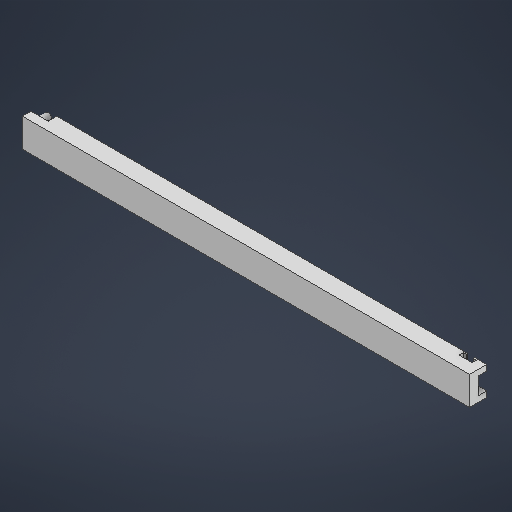
# Autodesk Inventor part: Wiper-supportipt
Saved by Autodesk Inventor 2026.2 (Build 302298010, 298A)
## iProperties
Created: 2026-06-02
Part Number: Wiper-supportipt
Material: Genérico
Document SubType Name: Modeling
Designer: pauli
Density: 1 g/cm^3
Appearance: Padrão
Author: pauli
Autodesk Inventor part; units mm, degrees
ref_plane "YZ Plane" through (0, 0, 0) normal (1, 0, 0) x (0, 1, 0)
ref_plane "XZ Plane" through (0, 0, 0) normal (0, 1, 0) x (-1, 0, 0)
ref_plane "XY Plane" through (0, 0, 0) normal (0, 0, 1) x (1, 0, 0)
sketch "Esboço1" plane through (0, 0, 0) normal (0, 0, 1) x (1, 0, 0)
  circle A0 centre (0, 0) radius 1.2
  line L0 (0, 0) -> (0, 4.75) construction
  circle A1 centre (0, 4.75) radius 1.2
  dimension "d0" = 2.4
  dimension "d1" = 4.75
  dimension "d2" = 2.4
  constraints: 2 centre point, 2 coincident, 2 end point, 1 vertical
  measures "d0" diameter of A0
  measures "d1" distance of L0.start L0.end
  measures "d2" diameter of A1
extrude "Extrusão1" add sketch "Esboço1" along normal blind 4
sketch "Esboço2" plane through (0, 4.75, 4) normal (0, 0, 1) x (1, 0, 0)
  circle A0 centre (0, -4.75) radius 1.2 projected
  line L0 (0, -4.75) -> (0, -2.375) construction
  line L1 (0, -2.375) -> (-2, -2.375) construction
  line L2 (-2, -2.375) -> (-2, 2.625)
  line L3 (-2, -2.375) -> (-2, -7.375)
  line L4 (-2, 2.625) -> (154.4, 2.625)
  line L5 (-2, -7.375) -> (154.4, -7.375)
  line L6 (154.4, -7.375) -> (154.4, 2.625)
  dimension "d9" = 2.375
  dimension "d10" = 2
  dimension "d11" = 5
  dimension "d12" = 5
  dimension "d13" = 156.4
  dimension "d14" = 156.4
  constraints: 14 end point, 3 vertical, 2 horizontal, 1 perpendicular
  measures "d9" distance of L0.start L0.end
  measures "d10" distance of L0.end L1.end
  measures "d11" distance of L1.end L2.end
  measures "d12" distance of L1.end L3.end
  measures "d13" distance of L2.end L4.end
  measures "d14" distance of L3.end L5.end
extrude "Extrusão2" add sketch "Esboço2" along normal blind 3 contours A0 | L2 L4 L6 L5 L3
sketch "Esboço3" plane through (0, 4.75, 4) normal (0, 0, -1) x (-1, 0, 0)
  circle A0 centre (0, 0) radius 1.2 projected
  line L0 (0, 0) -> (0, 2.625) construction
  line L1 (-154.4, 2.625) -> (2, 2.625) projected
  line L2 (0, 2.625) -> (-4, 2.625) construction
  line L3 (-4, 2.625) -> (-4, 0.625)
  line L4 (-4, 0.625) -> (-154.4, 0.625)
  line L5 (-154.4, 0.625) -> (-154.4, 2.625)
  line L6 (-154.4, 2.625) -> (-4, 2.625)
  line L7 (2, 2.625) -> (2, -7.375) projected
  line L8 (2, -2.375) -> (-158, -2.375) construction
  line L9 (-4, -7.375) -> (-4, -5.375)
  line L10 (-4, -5.375) -> (-154.4, -5.375)
  line L11 (-154.4, -5.375) -> (-154.4, -7.375)
  line L12 (-154.4, -7.375) -> (-4, -7.375)
  point P0 (0, -4.75)
  dimension "d19" = 4
  dimension "d20" = 2
  dimension "d21" = 150.4
  constraints: 22 end point, 4 symmetric about line, 2 point on line, 2 vertical, 1 collinear, 1 horizontal, 1 midpoint, 1 parallel, 1 perpendicular
  measures "d19" distance of L0.end L2.end
  measures "d20" distance of L2.end L3.end
  measures "d21" distance of L3.end L4.end
extrude "Extrusão3" add sketch "Esboço3" along normal blind 3 contours L1 L3 L4 L5 | L12 L11 L10 L9
sketch "Esboço4" plane through (-2, 7.375, 7) normal (0, 1, 0) x (1, 0, 0)
  line L0 (6, 3) -> (6, 6) projected
  line L1 (6, 4.5) -> (150.975, 4.5) construction
  line L2 (150.975, 4.5) -> (152.225, 4.5) construction
  line L3 (6, 3) -> (156.4, 3) projected
  line L4 (150.975, 4.5) -> (149.725, 4.5) construction
  line L5 (149.725, 5.5) -> (149.725, 6)
  line L6 (149.725, 6) -> (152.225, 6)
  line L7 (156.4, 6) -> (6, 6) projected
  line L8 (149.725, 6) -> (149.725, 5.5)
  line L9 (149.725, 5.5) -> (148.725, 5.5)
  line L10 (148.725, 5.5) -> (148.725, 4)
  line L11 (148.725, 4) -> (153.225, 4)
  line L12 (153.225, 4) -> (153.225, 5.5)
  line L13 (153.225, 5.5) -> (152.225, 5.5)
  line L14 (152.225, 5.5) -> (152.225, 6)
  point P0 (2, 7)
  point P1 (148.725, 4.5)
  point P2 (148.725, 3)
  point P3 (153.225, 3)
  dimension "d24" = 144.975
  dimension "d25" = 1.25
  dimension "d26" = 1.25
  dimension "d27" = 1
  dimension "d31" = 0.5
  dimension "d32" = 1.5
  dimension "d33" = 1
  dimension "d34" = 1.5
  dimension "d35" = 1
  dimension "d36" = 1
  dimension "d37" = 1
  dimension "d38" = 0.5
  constraints: 24 end point, 4 perpendicular, 4 point on line, 2 horizontal, 1 collinear, 1 midpoint, 1 parallel, 1 vertical
  measures "d24" distance of L1.start L1.end
  measures "d25" distance of L1.end L2.end
  measures "d26" distance of L1.end L4.end
  measures "d27" distance of L4.end point (148.725, 4.5)
  measures "d31" distance of L5.start L5.end
  measures "d32" distance of L9.end L10.end
  measures "d33" distance of L5.start L9.end
  measures "d34" distance of L11.end L12.end
  measures "d35" distance of L12.end L13.end
  measures "d36" distance of L9.end point (148.725, 4.5)
  measures "d37" distance of L13.end L2.end
  measures "d38" distance of L13.end L6.end
extrude "Extrusão4" cut sketch "Esboço4" against normal up to surface (10 mm away)
